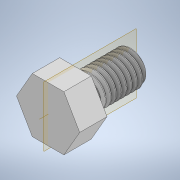
# Autodesk Inventor part: exBolt0_3-V01
Saved by Autodesk Inventor 2021.1 (Build 251245010, 245A)
## iProperties
Created: 2020-10-15
Part Number: exBolt0_3-V01
Material: Generic
Document SubType Name: Modeling
Designer: robst
Density: 1 g/cm^3
Appearance: Default
Author: robst
Autodesk Inventor part; units mm, degrees
ref_plane "XZ Plane" through (0, 0, 0) normal (0, 1, 0) x (-1, 0, 0)
ref_plane "XY Plane" through (0, 0, 0) normal (0, 0, 1) x (1, 0, 0)
sketch "Sketch1" plane through (0, 0, 0) normal (0, 0, 1) x (1, 0, 0)
  line L0 (-3.6662, 6.35) -> (3.6662, 6.35)
  line L1 (3.6662, 6.35) -> (7.3323, 0)
  line L2 (7.3323, 0) -> (3.6662, -6.35)
  line L3 (3.6662, -6.35) -> (-3.6662, -6.35)
  line L4 (-3.6662, -6.35) -> (-7.3323, 0)
  line L5 (-7.3323, 0) -> (-3.6662, 6.35)
  point P0 (0, 0)
  point P1 (0, 0)
  dimension "d0" = 12.7
  constraints: 12 end point, 1 coincident, 1 horizontal, 13 other
  measures "d0" distance between parallel lines of L3 L0
extrude "Extrusion1" add sketch "Sketch1" along normal blind 6.35
sketch "Sketch2" plane through (0, 0, 0) normal (0, 0, -1) x (-1, 0, 0)
  circle A0 centre (0, 0) radius 3.81
  dimension "d3" = 7.62
  constraints: 1 centre point, 1 coincident
  measures "d3" diameter of A0
extrude "Extrusion2" add sketch "Sketch2" along normal blind 12.7
sketch "Sketch4" plane through (0, 0, 0) normal (1, 0, 0) x (0, 1, 0)
  line L0 (3.81, 0) -> (3.81, -12.7) projected
  line L1 (-3.81, -12.7) -> (3.81, -12.7) projected
  line L2 (3.81, -13.9095) -> (3.81, -14.9229)
  line L3 (3.81, -14.9229) -> (3.1191, -14.524)
  line L4 (3.1191, -14.3084) -> (3.81, -13.9095)
  arc A0 (3.1191, -14.3084) -> (3.1191, -14.524) centre (3.1814, -14.4162) ccw
  line L5 (0, 0) -> (0, 6.35) construction
  line L6 (0, 0) -> (0, -12.7) construction
  dimension "d6" = 60
  dimension "d7" = 0.1245
  dimension "d8" = 1.2095
  dimension "d9" = 3.0569
  dimension "d10" = 3.81
  constraints: 8 end point, 2 point on circle, 2 tangent, 1 centre point, 1 collinear, 1 equal length, 1 midpoint, 1 vertical
  measures "d6" angle of L3 L4
  measures "d7" radius of A0
  measures "d8" distance of L2.start L0.end
  measures "d9" distance edge to line of A0 L6
  measures "d10" distance between parallel lines of L2 L6
coil "Coil1" sketch "Sketch4" operation cut axis through (0, 0, -10) along (0, 0, 1) pitch 1.2095 turns 12.25 hand right
equation "\"d3\" = a1Major"
equation "\"d7\" = a1RootRadius"
equation "\"d8\" = pitch"
equation "\"d9\" = a1MinorRadius"
equation "\"d11\" = pitch"
equation "\"a1Major\" = 7.62"
equation "\"a1Minor\" = 6.11378"
equation "\"a1RootRadius\" = 0.12446"
equation "\"a1MinorRadius\" = 0.5 * a1Minor"
equation "\"pitch\" = 1.209524"
body "Solid1"
